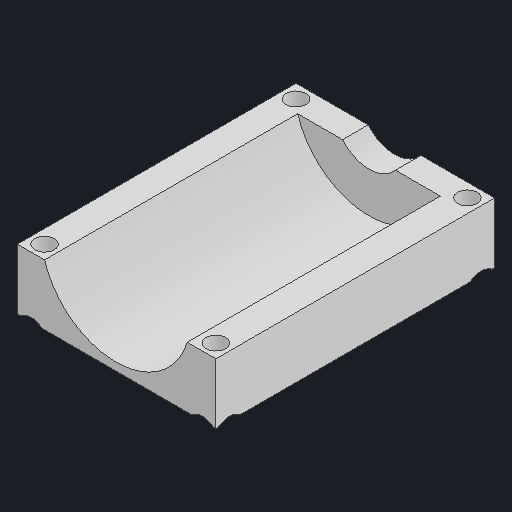
# Autodesk Inventor part: right_motor_mount_ceil
Saved by Autodesk Inventor 2023 (Build 270158000, 158)
## iProperties
Created: 2024-04-14
Part Number: right_motor_mount_ceil
Material: Generic
Document SubType Name: Modeling
Designer: szymo
Density: 1 g/cm^3
Appearance: Default
Author: szymo
Autodesk Inventor part; units mm, degrees
ref_plane "YZ Plane" through (0, 0, 0) normal (1, 0, 0) x (0, 1, 0)
sketch "Sketch1" plane through (0, 0, 0) normal (0, 0, 1) x (1, 0, 0)
  circle A0 centre (0, 0) radius 13.7 projected
  line L0 (18.375, 15.375) -> (-18.1, 15.375) projected
  line L1 (-18.1, 15.375) -> (-18.1, -4) projected
  line L2 (-18.1, -4) -> (-13.1031, -4) projected
  arc A1 (13.1031, -4) -> (-13.1031, -4) centre (0, 0) ccw projected
  line L3 (13.1031, -4) -> (18.375, -4) projected
  line L4 (18.375, -4) -> (18.375, 15.375) projected
  line L5 (18.375, -4) -> (-18.1, -4)
  line L6 (-18.1, -4) -> (-18.1, -15.125)
  line L7 (-18.1, -15.125) -> (18.375, -15.125)
  line L8 (18.375, -15.125) -> (18.375, -4)
  circle A2 centre (44.375, 8.875) radius 25 projected
  point P0 (0, -13.7)
  point P1 (44.375, -16.125)
  dimension "d2" = 29.075
  dimension "d15" = 1
  constraints: 8 end point, 2 parallel, 1 horizontal, 1 perpendicular, 1 point on circle, 1 vertical alignment, 1 other
  measures "d2" distance from line of L0 point (0, -13.7)
  measures "d15" distance from line of L7 point (44.375, -16.125)
ref_plane "Work Plane1" through (-13.7, -13.7, -46.5) normal (0, 0, -1) x (0, 1, 0)
extrude "Extrusion1" add sketch "Sketch1" against normal up to surface (46.5 mm away) contours A0 L3 L8 L7 L6 L2
sketch "Sketch2" plane through (18.375, -15.125, -46.5) normal (0, 0, -1) x (-1, 0, 0)
  circle A0 centre (26.375, 15.2) radius 1.0564 projected
  circle A1 centre (10.375, 15.2) radius 1.0564 projected
  circle A2 centre (18.375, 15.2) radius 5 projected
  circle A3 centre (18.375, 15.2) radius 13.7 projected
  arc A4 (23.2981, 11.2) -> (13.4519, 11.2) centre (18.375, 15.2) ccw projected
  circle A5 centre (18.375, 15.2) radius 6.3433
  line L0 (36.475, 0) -> (0, 0) projected
  line L1 (0, 11.125) -> (5.2719, 11.125) projected
  line L2 (36.475, 0) -> (0, 0)
  line L3 (0, 0) -> (0, 11.125)
  line L4 (0, 11.125) -> (36.475, 11.125)
  line L5 (36.475, 11.125) -> (36.475, 0)
  point P0 (18.375, 15.125)
  point P1 (23.2362, 11.125)
  point P2 (13.5138, 11.125)
  constraints: 8 end point, 2 parallel, 1 centre point, 1 coincident, 1 concentric, 1 horizontal, 1 perpendicular, 1 other
ref_plane "Work Plane2" through (-18.1, -4, -51.2) normal (0, 0, -1) x (0, 1, 0)
extrude "Extrusion2" add sketch "Sketch2" along normal up to surface (4.7 mm away) contours A5 L4 A3 | A3 L4 L5 L0 L3 L1
sketch "Sketch3" plane through (-18.1, -15.125, 0) normal (0, -1, 0) x (1, 0, 0)
  circle A0 centre (33.975, -2.5) radius 1.8 projected
  circle A1 centre (33.975, -48.7) radius 1.8 projected
  circle A2 centre (2.5, -48.7) radius 1.8 projected
  circle A3 centre (2.5, -2.5) radius 1.8 projected
  point P0 (18.1, 0)
  constraints: 4 coincident
hole "Hole1" at (15.875, -15.125, -2.5) at (15.875, -15.125, -48.7) at (-15.6, -15.125, -48.7) at (-15.6, -15.125, -2.5) direction (0, 1, 0) diameter 3.6 end through all countersink diameter 6.5 countersink angle 90 clearance for "Countersunk Flat Head Screw ISO 2009/7046" size "M3" standard "ISO"
body "Solid1"
